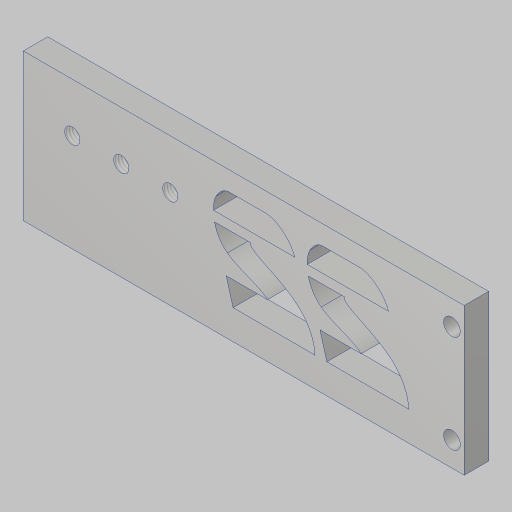
# Autodesk Inventor part: EL2-021
Saved by Autodesk Inventor 2023.5 (Build 275446000, 446)
## iProperties
Created: 2025-01-21
Part Number: EL2-021
Material: Aluminum 6061
Document SubType Name: Modeling
Designer: slick
Density: 2.7 g/cm^3
Appearance: Aluminum - Flat
Author: slick
Autodesk Inventor part; units mm, degrees
ref_plane "YZ Plane" through (0, 0, 0) normal (1, 0, 0) x (0, 1, 0)
ref_plane "XZ Plane" through (0, 0, 0) normal (0, 1, 0) x (-1, 0, 0)
ref_plane "XY Plane" through (0, 0, 0) normal (0, 0, 1) x (1, 0, 0)
sketch "Sketch1" plane through (0, 0, 0) normal (0, 0, 1) x (1, 0, 0)
  line L0 (57.15, -19.05) -> (-57.15, -19.05)
  line L1 (-57.15, -19.05) -> (-57.15, 19.05)
  line L2 (-57.15, 19.05) -> (57.15, 19.05)
  line L3 (57.15, 19.05) -> (57.15, -19.05)
  line L4 (57.15, -19.05) -> (-57.15, 19.05) construction
  line L5 (-57.15, -19.05) -> (57.15, 19.05) construction
  point P0 (0, 0)
  dimension "d0" = 114.3
  dimension "d1" = 38.1
  constraints: 12 end point, 2 midpoint, 2 parallel, 1 horizontal, 1 perpendicular
  measures "d0" distance of L1.end L2.end
  measures "d1" distance of L0.end L1.end
extrude "Extrusion1" add sketch "Sketch1" along normal blind 6.35
sketch "Sketch2" plane through (0, 0, 6.35) normal (0, 0, 1) x (1, 0, 0)
  line L0 (-57.15, 19.05) -> (-57.15, -19.05) projected
  line L1 (57.15, 19.05) -> (-57.15, 19.05) projected
  point P0 (0, 0)
  point P1 (-44.45, 6.35)
  point P2 (-31.75, 6.35)
  point P3 (-19.05, 6.35)
  point P4 (-57.15, 0)
  dimension "d5" = 12.7
  dimension "d6" = 12.7
  dimension "d14" = 12.7
  dimension "d15" = 12.7
  constraints: 2 horizontal alignment, 1 midpoint
  measures "d5" distance of point (-31.75, 6.35) point (-44.45, 6.35)
  measures "d6" distance of point (-31.75, 6.35) point (-19.05, 6.35)
  measures "d14" distance from line of L1 point (-44.45, 6.35)
  measures "d15" distance from line of L0 point (-44.45, 6.35)
hole "Hole1" at (-44.45, 6.35, 6.35) at (-31.75, 6.35, 6.35) at (-19.05, 6.35, 6.35) direction (0, 0, -1) diameter 3.9624 end through all thread size "10-32 UNF" class "2B" standard "ANSI Unified Screw Threads"
sketch "Sketch3" plane through (0, 0, 6.35) normal (0, 0, 1) x (1, 0, 0)
  line L0 (57.15, 19.05) -> (-57.15, 19.05) projected
  line L1 (-57.15, -19.05) -> (57.15, -19.05) projected
  line L2 (57.15, -19.05) -> (57.15, 19.05) projected
  point P0 (0, 0)
  point P1 (53.975, 12.7)
  point P2 (53.975, -12.7)
  dimension "d16" = 6.35
  dimension "d17" = 6.35
  dimension "d18" = 3.175
  constraints: 1 vertical alignment
  measures "d16" distance from line of L0 point (53.975, 12.7)
  measures "d17" distance from line of L1 point (53.975, -12.7)
  measures "d18" distance from line of L2 point (53.975, 12.7)
hole "Hole2" at (53.975, 12.7, 6.35) at (53.975, -12.7, 6.35) direction (0, 0, -1) diameter 4.318 end through all clearance for "Flat Head Machine Screw (82)" size "#8" standard "Ansi Unified Screw Threads"
sketch "Sketch4" plane through (0, 0, 0) normal (0, 0, -1) x (-1, 0, 0)
  line L0 (-42.3155, 14.0553) -> (6.0308, 14.0553) construction
  line L1 (6.0308, 14.0553) -> (6.0308, -14.8528) construction
  line L2 (6.0308, -14.8528) -> (-42.3155, -14.8528) construction
  line L3 (-42.3155, -14.8528) -> (-42.3155, 14.0553) construction
  line L4 (-42.7802, -11.4255) -> (-21.5429, -11.3851)
  line L5 (-21.5429, -11.3851) -> (-19.7647, -5.121)
  line L6 (-19.7647, -5.121) -> (-30.4541, -5.121)
  spline S0 degree 2 poles (-30.4541, -5.121) (-28.9184, -3.8277) (-21.5833, -0.9786) (-20.0678, 0.153) knots 0 0 0 1 2 2 2
  spline S1 degree 2 poles (-20.0678, 0.153) (-17.4409, 2.2141) (-16.7538, 5.4674) knots 0 0 0 1 1 1
  line L7 (-16.7538, 5.4674) -> (-26.0692, 5.4674)
  spline S2 degree 2 poles (-26.0692, 5.4674) (-26.0288, 5.3866) (-26.0288, 5.2856) knots 0 0 0 1 1 1
  spline S3 degree 2 poles (-26.0288, 5.2856) (-26.0288, 4.255) (-29.8681, 2.4364) knots 0 0 0 1 1 1
  spline S4 degree 2 poles (-29.8681, 2.4364) (-35.5462, -0.2107) (-37.87, -2.1708) knots 0 0 0 1 1 1
  spline S5 degree 2 poles (-37.87, -2.1708) (-42.4165, -5.9292) (-42.7802, -11.4255) knots 0 0 0 1 1 1
  spline S6 degree 2 poles (-16.4507, 7.9327) (-16.4507, 10.216) (-17.1782, 11.5093) knots 0 0 0 1 1 1
  spline S7 degree 2 poles (-17.1782, 11.5093) (-18.5927, 14.0553) (-20.6942, 14.0553) knots 0 0 0 1 1 1
  line L8 (-20.6942, 14.0553) -> (-29.7266, 14.0553)
  spline S8 degree 2 poles (-29.7266, 14.0553) (-32.1515, 14.0553) (-36.698, 10.3373) (-37.5063, 7.9327) knots 0 0 0 1 2 2 2
  line L9 (-37.5063, 7.9327) -> (-16.4507, 7.9327)
  line L10 (-18.4714, -11.4255) -> (2.766, -11.3851)
  line L11 (2.766, -11.3851) -> (4.5442, -5.121)
  line L12 (4.5442, -5.121) -> (-6.1452, -5.121)
  spline S9 degree 2 poles (-6.1452, -5.121) (-4.6095, -3.8277) (2.7256, -0.9786) (4.2411, 0.153) knots 0 0 0 1 2 2 2
  spline S10 degree 2 poles (4.2411, 0.153) (6.868, 2.2141) (7.555, 5.4674) knots 0 0 0 1 1 1
  line L13 (7.555, 5.4674) -> (-1.7604, 5.4674)
  spline S11 degree 2 poles (-1.7604, 5.4674) (-1.7199, 5.3866) (-1.7199, 5.2856) knots 0 0 0 1 1 1
  spline S12 degree 2 poles (-1.7199, 5.2856) (-1.7199, 4.255) (-5.5592, 2.4364) knots 0 0 0 1 1 1
  spline S13 degree 2 poles (-5.5592, 2.4364) (-11.2374, -0.2107) (-13.5612, -2.1708) knots 0 0 0 1 1 1
  spline S14 degree 2 poles (-13.5612, -2.1708) (-18.1077, -5.9292) (-18.4714, -11.4255) knots 0 0 0 1 1 1
  spline S15 degree 2 poles (7.8581, 7.9327) (7.8581, 10.216) (7.1306, 11.5093) knots 0 0 0 1 1 1
  spline S16 degree 2 poles (7.1306, 11.5093) (5.7162, 14.0553) (3.6147, 14.0553) knots 0 0 0 1 1 1
  line L14 (3.6147, 14.0553) -> (-5.4178, 14.0553)
  spline S17 degree 2 poles (-5.4178, 14.0553) (-7.8426, 14.0553) (-12.3892, 10.3373) (-13.1974, 7.9327) knots 0 0 0 1 2 2 2
  line L15 (-13.1974, 7.9327) -> (7.8581, 7.9327)
  point P0 (0, 0)
  constraints: 2 other
emboss "Emboss1" sketch "Sketch4" operation cut depth 6.35 direction (0, 0, 1)
equation "\"d5\" = d4"
equation "\"d6\" = d4"
equation "\"d4\" = 12.7"
body "Solid1"
